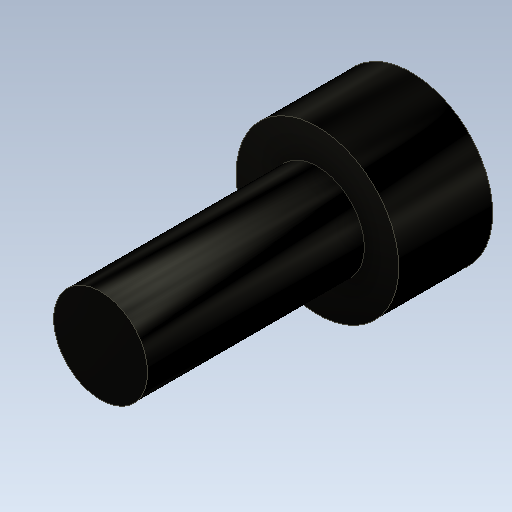
# Autodesk Inventor part: M2.6 ボルト 6mm
Saved by Autodesk Inventor 2020.2 (Build 242310000, 310)
## iProperties
Created: 2017-03-05
Part Number: M2.6 ボルト 6mm
Material: 鋼
Document SubType Name: Modeling
Designer: Takumi
Mass: 0.574675 g
Surface Area: 1.17574 cm^2
Volume: 0.073207 cm^3
Density: 7.85 g/cm^3
Appearance: ガンメタル
Author: Takumi
Autodesk Inventor part; units mm, degrees
ref_plane "YZ Plane" through (0, 0, 0) normal (1, 0, 0) x (0, 1, 0)
ref_plane "XZ Plane" through (0, 0, 0) normal (0, 1, 0) x (-1, 0, 0)
ref_plane "XY Plane" through (0, 0, 0) normal (0, 0, 1) x (1, 0, 0)
sketch "スケッチ1" plane through (0, 0, 0) normal (0, 0, 1) x (1, 0, 0)
  circle A0 centre (0, 0) radius 2.25
  dimension "d0" = 4.5
  constraints: 1 centre point, 1 coincident
  measures "d0" diameter of A0
extrude "押し出し1" add sketch "スケッチ1" along normal blind 2.6
sketch "スケッチ2" plane through (0, 0, 2.6) normal (0, 0, 1) x (1, 0, 0)
  circle A0 centre (0, 0) radius 1.3
  dimension "d3" = 2.6
  constraints: 1 centre point, 1 coincident
  measures "d3" diameter of A0
extrude "押し出し2" add sketch "スケッチ2" along normal blind 6
